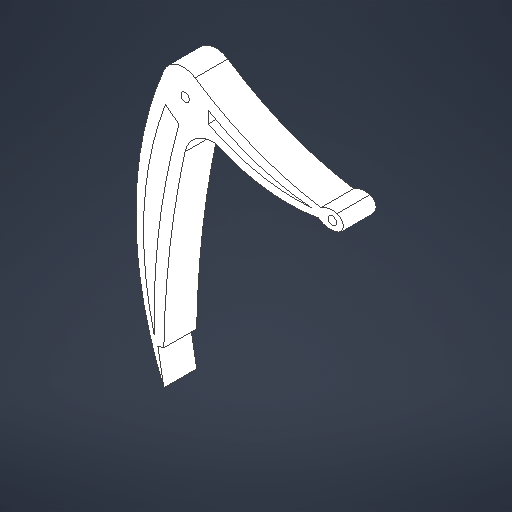
# Autodesk Inventor part: Claw
Saved by Autodesk Inventor 2026.1 (Build 301233020, 233B)
## iProperties
Created: 2025-11-27
Part Number: Claw
Material: Generic
Document SubType Name: Modeling
Designer: sarab
Density: 1 g/cm^3
Appearance: Default
Author: sarab
Autodesk Inventor part; units mm, degrees
ref_plane "YZ Plane" through (0, 0, 0) normal (1, 0, 0) x (0, 1, 0)
ref_plane "XZ Plane" through (0, 0, 0) normal (0, 1, 0) x (-1, 0, 0)
ref_plane "XY Plane" through (0, 0, 0) normal (0, 0, 1) x (1, 0, 0)
sketch "Sketch1" plane through (0, 0, 0) normal (0, 0, 1) x (1, 0, 0)
  circle A0 centre (-218.543, 11.2583) radius 1.841
  circle A1 centre (-155.8206, -2.8835) radius 1.841
  line L0 (-230.2092, -86.3504) -> (-227.6561, -85.8234)
  arc A2 (-218.6185, -8.9067) -> (-227.6561, -85.8234) centre (166.9594, -93.2007) ccw
  arc A3 (-205.5726, 0.7003) -> (-218.6185, -8.9067) centre (-206.6279, -11.5281) ccw
  arc A4 (-205.5726, 0.7003) -> (-161.7862, -4.929) centre (-174.5768, 68.6888) ccw
  arc A5 (-161.7862, -4.929) -> (-153.1858, -5.8609) centre (-156.6626, 2.2036) ccw
  arc A6 (-153.1858, -5.8609) -> (-153.782, 0.6635) centre (-154.5502, -2.6961) ccw
  arc A7 (-153.782, 0.6635) -> (-160.6438, -0.507) centre (-155.9827, -7.1338) ccw
  arc A8 (-214.3232, 20.5519) -> (-160.6438, -0.507) centre (-140.3024, 130.2877) ccw
  arc A9 (-214.3232, 20.5519) -> (-227.6561, 16.6026) centre (-219.3619, 13.0819) ccw
  arc A10 (-227.6561, 16.6026) -> (-227.6561, -100.5779) centre (-89.6281, -41.9876) ccw
  line L1 (-227.6561, -100.5779) -> (-230.2092, -86.3504)
  point P0 (0, 0)
  point P1 (-190.934, -110.2879)
  constraints: 18 point on circle, 11 centre point, 4 end point
extrude "Extrusion1" add sketch "Sketch1" along normal blind 14
sketch "Sketch2" plane through (0, 0, 14) normal (0, 0, 1) x (1, 0, 0)
  arc A0 (-226.9928, 4.3779) -> (-231.786, -82.917) centre (-90.6456, -46.8878) ccw
  arc A1 (-221.1828, 0) -> (-231.786, -82.917) centre (55.5969, -77.5303) ccw
  line L0 (-226.9928, 4.3779) -> (-221.1828, 0)
  arc A2 (-208.6913, 11.3499) -> (-164.5355, -2.5941) centre (-156.1757, 100.764) ccw
  arc A3 (-208.6913, 6.3406) -> (-164.5355, -2.5941) centre (-170.8567, 79.7445) ccw
  line L1 (-208.6913, 11.3499) -> (-208.6913, 6.3406)
  point P0 (0, 0)
  constraints: 8 point on circle, 4 centre point, 4 end point, 1 vertical
extrude "Extrusion2" cut sketch "Sketch2" against normal blind 14
body "Solid1"
